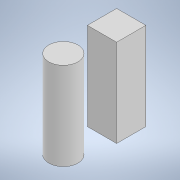
# Autodesk Inventor part: pegs
Saved by Autodesk Inventor 2021 (Build 250183000, 183)
## iProperties
Created: 2020-05-07
Part Number: pegs
Material: Generic
Document SubType Name: Modeling
Designer: david
Density: 1 g/cm^3
Appearance: Default
Author: david
Autodesk Inventor part; units mm, degrees
ref_plane "YZ Plane" through (0, 0, 0) normal (1, 0, 0) x (0, 1, 0)
ref_plane "XZ Plane" through (0, 0, 0) normal (0, 1, 0) x (-1, 0, 0)
ref_plane "XY Plane" through (0, 0, 0) normal (0, 0, 1) x (1, 0, 0)
sketch "Sketch1" plane through (0, 0, 0) normal (0, 1, 0) x (-1, 0, 0)
  line L0 (40.5057, -117.9366) -> (91.3057, -117.9366)
  line L1 (91.3057, -117.9366) -> (91.3057, -168.7366)
  line L2 (91.3057, -168.7366) -> (40.5057, -168.7366)
  line L3 (40.5057, -168.7366) -> (40.5057, -117.9366)
  circle A0 centre (69.9339, -54.8282) radius 25.4
  point P0 (0, 0)
  dimension "d0" = 50.8
  dimension "d1" = 50.8
  dimension "d2" = 50.8
  constraints: 8 end point, 2 parallel, 1 centre point, 1 horizontal, 1 perpendicular
  measures "d0" distance of L0.end L1.end
  measures "d1" distance of L1.end L2.end
  measures "d2" diameter of A0
extrude "Extrusion1" add sketch "Sketch1" along normal blind 152.4
body "Solid1"
